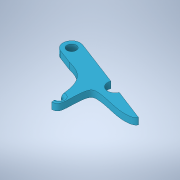
# Autodesk Inventor part: Springy
Saved by Autodesk Inventor 2020.1 (Build 241239000, 239)
## iProperties
Created: 2019-07-20
Part Number: Springy
Material: Generic
Document SubType Name: Modeling
Designer: Petar
Density: 1 g/cm^3
Appearance: Turquoise
Mass: 1.03312 g
Surface Area: 11.2986 cm^2
Volume: 1.03312 cm^3
Author: Petar
Autodesk Inventor part; units mm, degrees
ref_plane "YZ Plane" through (0, 0, 0) normal (1, 0, 0) x (0, 1, 0)
ref_plane "XZ Plane" through (0, 0, 0) normal (0, 1, 0) x (-1, 0, 0)
ref_plane "XY Plane" through (0, 0, 0) normal (0, 0, 1) x (1, 0, 0)
sketch "Sketch1" plane through (0, 0, 0) normal (0, 1, 0) x (-1, 0, 0)
  circle A0 centre (16.7493, -22.6165) radius 2.15
  arc A1 (-5.747, -18.3073) -> (-12.253, -15.726) centre (-9.0167, -17.0587) ccw
  line L0 (16.7493, -22.6165) -> (-9.0167, -17.0587) construction
  circle A2 centre (-20.45, 0) radius 2
  line L1 (16.7493, -22.6165) -> (-20.45, 0) construction
  arc A3 (15.3223, -26.3533) -> (18.1763, -18.8797) centre (16.7493, -22.6165) ccw
  line L2 (18.1763, -18.8797) -> (11.637, -16.3824)
  line L3 (-9.0167, -17.0587) -> (-20.45, 0) construction
  line L4 (15.3223, -26.3533) -> (-5.747, -18.3073)
  line L5 (0, 0) -> (41.7929, 0) construction
  arc A4 (-20.45, 0) -> (-26.74, -20.6222) centre (16.7493, -22.6165) ccw construction
  line L6 (-31.9548, -27.9305) -> (-25.3775, -10.864) construction
  arc A5 (-0.1379, 1.192) -> (0.1379, -1.192) centre (0, 0) ccw
  line L7 (11.637, -16.3824) -> (10.1158, -15.8015) construction
  line L8 (10.1158, -15.8015) -> (1.6573, -14.7272) construction
  line L9 (1.6573, -14.7272) -> (0.9757, -8.4344) construction
  line L10 (0.9757, -8.4344) -> (0.1379, -1.192) construction
  spline S0 degree 4 poles (11.637, -16.3824) (10.1158, -15.8015) (1.6573, -14.7272) (0.9757, -8.4344) (0.1379, -1.192) knots 1 1 1 1 1 2 2 2 2 2
  line L11 (0.1379, -1.192) -> (-0.1379, 1.192) construction
  line L12 (-0.1379, 1.192) -> (-0.4367, 3.7748)
  line L13 (-20.45, 0) -> (0, 0) construction
  line L14 (-0.4367, 3.7748) -> (-2.463, 3.5404) construction
  line L15 (-2.463, 3.5404) -> (-3.0764, 2.02) construction
  line L16 (-3.0764, 2.02) -> (-3.317, 0) construction
  line L17 (-3.317, 0) -> (-3.317, -2.3302) construction
  line L18 (-3.317, -2.3302) -> (-3.4686, -4.784) construction
  line L19 (-3.4686, -4.784) -> (-3.6938, -8.4307) construction
  line L20 (-3.6938, -8.4307) -> (-4.5575, -10.4149) construction
  line L21 (-4.5575, -10.4149) -> (-5.8935, -11.2504) construction
  line L22 (-5.8935, -11.2504) -> (-13.9739, -9.9274) construction
  line L23 (-13.9739, -9.9274) -> (-19.6159, -8.0541) construction
  line L24 (-19.6159, -8.0541) -> (-26.0225, -8.3663) construction
  line L25 (-26.0225, -8.3663) -> (-26.7114, -10.1539) construction
  spline S1 degree 4 poles (-0.4367, 3.7748) (-2.463, 3.5404) (-3.0764, 2.02) (-3.317, 0) (-3.317, -2.3302) (-3.4686, -4.784) (-3.6938, -8.4307) (-4.5575, -10.4149) (-5.8935, -11.2504) (-13.9739, -9.9274) (-19.6159, -8.0541) (-26.0225, -8.3663) (-26.7114, -10.1539) knots 0 0 0 0 0 1 2 3 4 5 6 7 8 9 9 9 9 9
  line L26 (16.7493, -22.6165) -> (7.1033, -18.9328) construction
  line L27 (-26.7114, -10.1539) -> (-12.253, -15.726)
  dimension "d1" = 7
  dimension "d2" = 26.3586
  dimension "d3" = 4
  dimension "d4" = 43.535
  dimension "d5" = 4
  dimension "d6" = 20.5358
  dimension "d7" = 7
  dimension "d9" = 1.5
  dimension "d10" = 1.2
  dimension "d21" = 17.25
  dimension "d22" = 2.6
  dimension "d23" = 117.5
  dimension "d24" = 4.3
  constraints: 24 end point, 10 point on circle, 6 centre point, 4 tangent, 2 coincident, 2 horizontal, 2 parallel, 2 point on line, 1 collinear, 1 midpoint, 1 perpendicular, 12 other
  measures "d1" diameter of A1
  measures "d2" distance of L0.start L0.end
  measures "d3" diameter of A2
  measures "d4" distance of L0.start L1.end
  measures "d5" radius of A3
  measures "d6" distance of L0.end L1.end
  measures "d7" distance of L2.start L2.end
  measures "d9" distance from line of L25.end L6
  measures "d10" radius of A5
  measures "d22" distance of L11.end L12.end
  measures "d23" angle of L11 L26
  measures "d24" diameter of A0
extrude "Extrusion1" add sketch "Sketch1" along normal blind 3 contours A1 L27 S1 L12 A5 S0 L2 A3 L4
fillet "Fillet3" radius 1.5 2 edges at (1.192, 3, -0.1379) (1.192, 0, -0.1379)
ref_plane "Work Plane1" through (0, 1.5, 0) normal (0, 1, 0) x (1, 0, 0)
ref_plane "Work Plane2" through (20.45, 0, 0) normal (0, 0, 1) x (-1, 0, 0)
sketch "Sketch3" plane through (20.45, 0, 0) normal (0, 0, 1) x (-1, 0, 0)
  arc A0 (17.75, -3) -> (17.75, 0) centre (17.75, -1.5) ccw projected
  point P0 (20.45, 0)
body "Solid1"
